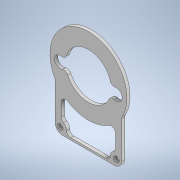
# Autodesk Inventor part: Thrust_spacer_01
Saved by Autodesk Inventor 2020.4 (Build 244396000, 396)
## iProperties
Created: 2021-09-22
Part Number: Thrust_spacer_01
Material: 一般
Document SubType Name: Modeling
Designer: Masato
Density: 1 g/cm^3
Appearance: 既定
Author: Masato
Autodesk Inventor part; units mm, degrees
ref_plane "YZ Plane" through (0, 0, 0) normal (1, 0, 0) x (0, 1, 0)
ref_plane "XZ Plane" through (0, 0, 0) normal (0, 1, 0) x (-1, 0, 0)
ref_plane "XY Plane" through (0, 0, 0) normal (0, 0, 1) x (1, 0, 0)
derived "Trunk_horizontal_frame_01.ipt"
sketch "スケッチ1" plane through (0, 0, 0) normal (0, 0, 1) x (1, 0, 0)
  line L0 (-62.5, 30.75) -> (62.5, 30.75)
  line L1 (62.5, 30.75) -> (62.5, -30.75)
  line L2 (62.5, -30.75) -> (-62.5, -30.75)
  line L3 (-62.5, -30.75) -> (-62.5, 30.75)
  line L4 (-62.5, 30.75) -> (62.5, -30.75) construction
  line L5 (62.5, 30.75) -> (-62.5, -30.75) construction
  line L6 (-62.5, 2.25) -> (62.5, 2.25) construction
  circle A0 centre (-44, 2.25) radius 18.5 construction
  line L7 (-62.5, 0) -> (62.5, 0) construction
  line L8 (0, 30.75) -> (0, -30.75) construction
  circle A1 centre (-44, 2.25) radius 10.5 construction
  line L9 (-57.5, 1.25) -> (-30.5, 1.25) construction
  line L10 (-30.5, 1.25) -> (-30.5, -25.75) construction
  line L11 (-30.5, -25.75) -> (-57.5, -25.75) construction
  line L12 (-57.5, -25.75) -> (-57.5, 1.25) construction
  line L13 (-44, 1.25) -> (-44, -25.75) construction
  line L14 (-57.5, -12.25) -> (-30.5, -12.25) construction
  circle A2 centre (-57.5, 1.25) radius 1.35
  circle A3 centre (-57.5, -25.75) radius 1.35
  circle A4 centre (-30.5, 1.25) radius 1.35
  circle A5 centre (-30.5, -25.75) radius 1.35
  line L15 (-28, 21.75) -> (-23, 21.75) construction
  line L16 (-23, 21.75) -> (-23, 11.75) construction
  line L17 (-23, 11.75) -> (-28, 11.75) construction
  line L18 (-28, 11.75) -> (-28, 21.75) construction
  line L19 (-28, 21.75) -> (-23, 11.75) construction
  line L20 (-23, 21.75) -> (-28, 11.75) construction
  line L21 (-28.01, 21.76) -> (-22.99, 21.76)
  line L22 (-22.99, 21.76) -> (-22.99, 11.74)
  line L23 (-22.99, 11.74) -> (-28.01, 11.74)
  line L24 (-28.01, 11.74) -> (-28.01, 21.76)
  line L25 (-28.01, 21.76) -> (-22.99, 11.74) construction
  line L26 (-22.99, 21.76) -> (-28.01, 11.74) construction
  line L27 (-28.01, 16.75) -> (-22.99, 16.75) construction
  line L28 (-25.5, 21.76) -> (-25.5, 11.74) construction
  arc A6 (-28.01, 21.76) -> (-28.01, 19.66) centre (-28.01, 20.71) ccw
  arc A7 (-22.99, 19.66) -> (-22.99, 21.76) centre (-22.99, 20.71) ccw
  arc A8 (-22.99, 11.74) -> (-22.99, 13.84) centre (-22.99, 12.79) ccw
  arc A9 (-28.01, 13.84) -> (-28.01, 11.74) centre (-28.01, 12.79) ccw
  circle A10 centre (-25.5, 27.75) radius 1.55
  arc A11 (-28.01, -19.66) -> (-28.01, -21.76) centre (-28.01, -20.71) ccw
  line L29 (-23, -21.75) -> (-28, -21.75) construction
  line L30 (-22.99, -21.76) -> (-28.01, -21.76)
  arc A12 (-22.99, -21.76) -> (-22.99, -19.66) centre (-22.99, -20.71) ccw
  line L31 (-28, -21.75) -> (-28, -9.25) construction
  line L32 (-28.01, -21.76) -> (-28.01, -9.24)
  line L33 (-28.01, -15.5) -> (-22.99, -15.5) construction
  line L34 (-25.5, -9.24) -> (-25.5, -21.76) construction
  line L35 (-28, -9.25) -> (-23, -21.75) construction
  line L36 (-23, -9.25) -> (-28, -21.75) construction
  line L37 (-28.01, -9.24) -> (-22.99, -21.76) construction
  line L38 (-22.99, -9.24) -> (-28.01, -21.76) construction
  line L39 (-23, -9.25) -> (-23, -21.75) construction
  line L40 (-22.99, -9.24) -> (-22.99, -21.76)
  circle A13 centre (-25.5, -27.75) radius 1.55
  arc A14 (-22.99, -11.34) -> (-22.99, -9.24) centre (-22.99, -10.29) ccw
  line L41 (-28, -9.25) -> (-23, -9.25) construction
  line L42 (-28.01, -9.24) -> (-22.99, -9.24)
  arc A15 (-28.01, -9.24) -> (-28.01, -11.34) centre (-28.01, -10.29) ccw
  circle A16 centre (-44, 2.25) radius 11
  arc A17 (-54.9991, 2.3936) -> (-54.8579, 0.4874) centre (-57.5, 1.25) ccw
  arc A18 (-33.1421, 0.4874) -> (-33.0009, 2.3936) centre (-30.5, 1.25) ccw
  circle A19 centre (30.5, 1.25) radius 1.35
  line L43 (57.5, 1.25) -> (30.5, 1.25) construction
  arc A20 (33.0009, 2.3936) -> (33.1421, 0.4874) centre (30.5, 1.25) ccw
  circle A21 centre (44, 2.25) radius 18.5 construction
  line L44 (62.5, 0) -> (-62.5, 0) construction
  line L45 (-62.5, 30.75) -> (62.5, -30.75) construction
  line L46 (62.5, 30.75) -> (-62.5, -30.75) construction
  line L47 (62.5, 2.25) -> (-62.5, 2.25) construction
  arc A22 (54.8579, 0.4874) -> (54.9991, 2.3936) centre (57.5, 1.25) ccw
  arc A23 (28.01, -11.34) -> (28.01, -9.24) centre (28.01, -10.29) ccw
  circle A24 centre (57.5, 1.25) radius 1.35
  circle A25 centre (44, 2.25) radius 10.5 construction
  circle A26 centre (44, 2.25) radius 11
  line L48 (57.5, -12.25) -> (30.5, -12.25) construction
  line L49 (57.5, -25.75) -> (57.5, 1.25) construction
  line L50 (30.5, 1.25) -> (30.5, -25.75) construction
  line L51 (44, 1.25) -> (44, -25.75) construction
  line L52 (30.5, -25.75) -> (57.5, -25.75) construction
  arc A27 (28.01, 11.74) -> (28.01, 13.84) centre (28.01, 12.79) ccw
  line L53 (23, 11.75) -> (28, 11.75) construction
  line L54 (22.99, 11.74) -> (28.01, 11.74)
  arc A28 (22.99, 13.84) -> (22.99, 11.74) centre (22.99, 12.79) ccw
  line L55 (28.01, 16.75) -> (22.99, 16.75) construction
  line L56 (25.5, 21.76) -> (25.5, 11.74) construction
  line L57 (28.01, 11.74) -> (28.01, 21.76)
  line L58 (22.99, 21.76) -> (28.01, 11.74) construction
  line L59 (22.99, 21.76) -> (22.99, 11.74)
  line L60 (28.01, 21.76) -> (22.99, 11.74) construction
  line L61 (23, 21.75) -> (23, 11.75) construction
  line L62 (28, 21.75) -> (23, 11.75) construction
  line L63 (28, 11.75) -> (28, 21.75) construction
  line L64 (23, 21.75) -> (28, 11.75) construction
  arc A29 (22.99, 21.76) -> (22.99, 19.66) centre (22.99, 20.71) ccw
  line L65 (28, 21.75) -> (23, 21.75) construction
  arc A30 (28.01, 19.66) -> (28.01, 21.76) centre (28.01, 20.71) ccw
  circle A31 centre (57.5, -25.75) radius 1.35
  line L66 (28, -9.25) -> (23, -9.25) construction
  line L67 (28.01, -9.24) -> (22.99, -9.24)
  arc A32 (22.99, -9.24) -> (22.99, -11.34) centre (22.99, -10.29) ccw
  line L68 (28.01, -15.5) -> (22.99, -15.5) construction
  line L69 (22.99, -9.24) -> (22.99, -21.76)
  line L70 (28.01, -9.24) -> (22.99, -21.76) construction
  line L71 (28.01, -21.76) -> (28.01, -9.24)
  line L72 (22.99, -9.24) -> (28.01, -21.76) construction
  line L73 (25.5, -9.24) -> (25.5, -21.76) construction
  line L74 (28, -21.75) -> (28, -9.25) construction
  line L75 (23, -9.25) -> (28, -21.75) construction
  line L76 (23, -9.25) -> (23, -21.75) construction
  line L77 (28, -9.25) -> (23, -21.75) construction
  arc A33 (22.99, -19.66) -> (22.99, -21.76) centre (22.99, -20.71) ccw
  arc A34 (28.01, -21.76) -> (28.01, -19.66) centre (28.01, -20.71) ccw
  line L78 (23, -21.75) -> (28, -21.75) construction
  circle A35 centre (30.5, -25.75) radius 1.35
  circle A36 centre (25.5, -27.75) radius 1.55
  line L79 (22.99, -21.76) -> (28.01, -21.76)
  circle A37 centre (25.5, 27.75) radius 1.55
  line L80 (28.01, 21.76) -> (22.99, 21.76)
  arc A38 (-44, -11.75) -> (-31.01, -2.9711) centre (-44, 2.25) ccw
  arc A39 (-55.2639, -27.75) -> (-56.99, -22.7937) centre (-57.5, -25.75) ccw
  line L81 (-56.99, -22.7937) -> (-56.99, -2.9711)
  line L82 (-55.2639, -27.75) -> (-32.7361, -27.75)
  arc A40 (-31.01, -22.7937) -> (-32.7361, -27.75) centre (-30.5, -25.75) ccw
  line L83 (-31.01, -22.7937) -> (-31.01, -2.9711)
  arc A41 (-56.99, -2.9711) -> (-44, -11.75) centre (-44, 2.25) ccw
  line L84 (56.99, -22.7937) -> (56.99, -2.9711)
  arc A42 (44, -11.75) -> (56.99, -2.9711) centre (44, 2.25) ccw
  arc A43 (31.01, -2.9711) -> (44, -11.75) centre (44, 2.25) ccw
  line L85 (31.01, -22.7937) -> (31.01, -2.9711)
  line L86 (55.2639, -27.75) -> (32.7361, -27.75)
  arc A44 (32.7361, -27.75) -> (31.01, -22.7937) centre (30.5, -25.75) ccw
  arc A45 (56.99, -22.7937) -> (55.2639, -27.75) centre (57.5, -25.75) ccw
  line L87 (-60, 14.25) -> (-28, 14.25) construction
  line L88 (-28, 14.25) -> (-28, -28.75) construction
  line L89 (-28, -28.75) -> (-60, -28.75) construction
  line L90 (-60, -28.75) -> (-60, 14.25) construction
  line L91 (-60, 14.25) -> (-28, -28.75) construction
  line L92 (-28, 14.25) -> (-60, -28.75) construction
  arc A46 (-54.583, 14.25) -> (-60, 2.25) centre (-44, 2.25) ccw construction
  arc A47 (-28, 2.25) -> (-33.417, 14.25) centre (-44, 2.25) ccw construction
  line L93 (-28, 30.75) -> (-62.5, 13.7615)
  line L94 (28, 30.75) -> (62.5, 13.7615)
  line L95 (-31.01, 25.9238) -> (-43.143, 19.9493)
  arc A48 (-56.99, -2.9711) -> (-56.1, -4.792) centre (-44, 2.25) ccw
  arc A49 (-43.143, 19.9493) -> (-42.477, 16.1669) centre (-42.2595, 18.155) ccw
  line L96 (-31.01, 14.25) -> (-36.7889, 14.25)
  arc A50 (-36.7889, 14.25) -> (-42.477, 16.1669) centre (-44, 2.25) ccw
  line L97 (-31.01, 14.25) -> (-31.01, 25.9238)
  line L98 (31.01, 25.9238) -> (43.143, 19.9493)
  line L99 (31.01, 14.25) -> (31.01, 25.9238)
  line L100 (31.01, 14.25) -> (36.7889, 14.25)
  arc A51 (42.477, 16.1669) -> (36.7889, 14.25) centre (44, 2.25) ccw
  arc A52 (42.477, 16.1669) -> (43.143, 19.9493) centre (42.2595, 18.155) ccw
  line L101 (-60, -7.0371) -> (-60, -25.3036)
  line L102 (-31.4464, -28.75) -> (-56.5536, -28.75)
  line L103 (-28, -25.3036) -> (-28, -7.0371)
  arc A53 (-28, -7.0371) -> (-60, -7.0371) centre (-44, 2.25) ccw
  arc A54 (-56.99, -10.9223) -> (-31.01, -10.9223) centre (-44, 2.25) ccw
  circle A55 centre (-25.5, -27.75) radius 2.75 construction
  arc A56 (-31.4464, -28.75) -> (-28, -25.3036) centre (-31.4464, -25.3036) ccw
  circle A57 centre (-30.5, -25.75) radius 2.4 construction
  arc A58 (-60, -25.3036) -> (-56.5536, -28.75) centre (-56.5536, -25.3036) ccw
  point P0 (0, 0)
  point P1 (-25.5, 16.75)
  point P2 (-25.5, -15.5)
  point P3 (25.5, 16.75)
  point P4 (25.5, -15.5)
  point P5 (-44, -7.25)
  point P6 (-28, -21.76)
  point P7 (-28, -9.24)
  point P8 (-33.0009, 2.3936)
  point P9 (-33.1421, 0.4874)
  point P10 (-28.1232, 11.7461)
  point P11 (-29.014, 13.0975)
  point P12 (-62.5, 2.25)
  point P13 (-52.1726, 18.8469)
  dimension "d5" = 5.5
  dimension "d8" = 4.8
  measures "d5" diameter of A55
  measures "d8" diameter of A57
extrude "押し出し1" add sketch "スケッチ1" along normal blind 1.5 contours A53 L95 A49 A50 L96 L97 A9 L103 L42 A15 L32 A11 L30 A56 L102 A58 L101 | A53 L97 L96 A50 A49 L95 | A53 A9 | L103 L30 L32 L42 | L32 A15 | A11 L32 | A38 L83 A54 L81 A41
fillet "フィレット1" radius 2 12 edges at (-28, -7.0371, 0.75) (-60, -7.0371, 0.75) (-56.99, -10.9223, 0.75) (-31.01, -10.9223, 0.75) (-31.01, -22.7937, 0.75) (-32.7361, -27.75, 0.75) (-55.2639, -27.75, 0.75) (-56.99, -22.7937, 0.75) (-54.8579, 0.4874, 0.75) (-54.9991, 2.3936, 0.75) (-33.0009, 2.3936, 0.75) (-33.1421, 0.4874, 0.75)
